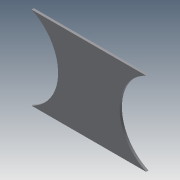
# Autodesk Inventor part: sablona_vystuha_clanek(1)
Saved by Autodesk Inventor 2013 (Build 170138000, 138)
## iProperties
Created: 2013-06-26
Part Number: sablona_vystuha_clanek(1)
Material: Generic
Document SubType Name: Modeling
Designer: idle-rug
Density: 1 g/cm^3
Author: idle-rug
Autodesk Inventor part; units mm, degrees
ref_plane "YZ Plane" through (0, 0, 0) normal (1, 0, 0) x (0, 1, 0)
ref_plane "XZ Plane" through (0, 0, 0) normal (0, 1, 0) x (-1, 0, 0)
ref_plane "XY Plane" through (0, 0, 0) normal (0, 0, 1) x (1, 0, 0)
sketch "Sketch1" plane through (0, 0, 0) normal (0, 1, 0) x (-1, 0, 0)
  line L0 (-50, -36.3) -> (50, -36.3)
  line L1 (50, 36.3) -> (-50, 36.3)
  line L2 (-50, -36.3) -> (50, 36.3) construction
  line L3 (50, -36.3) -> (-50, 36.3) construction
  arc A0 (50, 36.3) -> (50, -36.3) centre (66.8021, 0) ccw
  arc A1 (-50, -36.3) -> (-50, 36.3) centre (-66.8021, 0) ccw
  point P0 (0, 0)
  dimension "d0" = 100
  dimension "d1" = 72.6
  dimension "d4" = 40
  dimension "d5" = 40
  constraints: 8 end point, 4 point on circle, 2 centre point, 2 midpoint, 1 horizontal, 1 parallel
  measures "d0" distance of L1.end L1.start
  measures "d1" distance of L1.start L0.end
  measures "d4" radius of A0
  measures "d5" radius of A1
extrude "Extrusion1" add sketch "Sketch1" along normal blind 2
body "Solid1"
